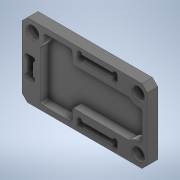
# Autodesk Inventor part: Cockpit_horizontal_frame_06
Saved by Autodesk Inventor 2020 (Build 240168000, 168)
## iProperties
Created: 2021-08-14
Part Number: Cockpit_horizontal_frame_06
Material: アセタール樹脂、黒
Document SubType Name: Modeling
Designer: Masato
Density: 1.425 g/cm^3
Appearance: 滑らか - 黒
Mass: 7.86831 g
Surface Area: 61.8804 cm^2
Volume: 5.52162 cm^3
d0: 59.500 mm
d1: 35.000 mm
d4: 18.833 mm
d6: 18.833 mm
d7: 0.050 mm
d8: 0.050 mm
d9: 1.050 mm
d15: 5.000 mm
d16: 0.00 deg
d17: 2.000 mm
d18: 0.00 deg
d23: 2.500 mm
d26: 35.750 mm
d27: 5.000 mm
d31: 3.200 mm
d32: 6.000 mm
d33: 5.000 mm
d34: 10.000 mm
Author: Masato
Autodesk Inventor part; units mm, degrees
ref_plane "YZ Plane" through (0, 0, 0) normal (1, 0, 0) x (0, 1, 0)
ref_plane "XZ Plane" through (0, 0, 0) normal (0, 1, 0) x (-1, 0, 0)
ref_plane "XY Plane" through (0, 0, 0) normal (0, 0, 1) x (1, 0, 0)
sketch "スケッチ1" plane through (0, 0, 0) normal (0, 0, 1) x (1, 0, 0)
  line L0 (29.75, 17.5) -> (29.75, -17.5)
  line L1 (29.75, -17.5) -> (-29.75, -17.5)
  line L2 (-29.75, -17.5) -> (-29.75, 17.5)
  line L3 (-29.75, 17.5) -> (29.75, -17.5) construction
  line L4 (29.75, 17.5) -> (-29.75, -17.5) construction
  line L5 (-3.4667, -15.05) -> (-1.3667, -15.05) construction
  line L6 (15.4667, -15.05) -> (15.4667, -12.45)
  line L7 (15.4667, -12.45) -> (13.3667, -12.45) construction
  line L8 (-3.4667, -12.45) -> (-3.4667, -15.05)
  line L9 (-3.4667, -15.05) -> (15.4667, -12.45) construction
  line L10 (15.4667, -15.05) -> (-3.4667, -12.45) construction
  line L11 (-3.4167, -12.5) -> (15.4167, -12.5) construction
  line L12 (15.4167, -12.5) -> (15.4167, -15) construction
  line L13 (15.4167, -15) -> (-3.4167, -15) construction
  line L14 (-3.4167, -15) -> (-3.4167, -12.5) construction
  line L15 (-3.4167, -12.5) -> (15.4167, -15) construction
  line L16 (15.4167, -12.5) -> (-3.4167, -15) construction
  arc A0 (-1.3667, -12.45) -> (-3.4667, -12.45) centre (-2.4167, -12.45) ccw
  line L17 (-3.4667, -13.75) -> (15.4667, -13.75) construction
  arc A1 (-3.4667, -15.05) -> (-1.3667, -15.05) centre (-2.4167, -15.05) ccw
  line L18 (-1.3667, -12.45) -> (-3.4667, -12.45) construction
  line L19 (-1.3667, -15.05) -> (13.3667, -15.05)
  line L20 (13.3667, -12.45) -> (-1.3667, -12.45)
  line L21 (13.3667, -15.05) -> (15.4667, -15.05) construction
  line L22 (-29.75, 17.5) -> (29.75, 17.5)
  line L23 (6, 17.5) -> (6, -17.5) construction
  line L24 (-29.75, 0) -> (29.75, 0) construction
  arc A2 (15.4667, -12.45) -> (13.3667, -12.45) centre (14.4167, -12.45) ccw
  arc A3 (13.3667, -15.05) -> (15.4667, -15.05) centre (14.4167, -15.05) ccw
  line L25 (-3.4667, 15.05) -> (-1.3667, 15.05) construction
  line L26 (15.4667, 15.05) -> (15.4667, 12.45)
  line L27 (15.4667, 12.45) -> (13.3667, 12.45) construction
  line L28 (-3.4667, 12.45) -> (-3.4667, 15.05)
  line L29 (-3.4667, 15.05) -> (15.4667, 12.45) construction
  line L30 (15.4667, 15.05) -> (-3.4667, 12.45) construction
  line L31 (-3.4167, 12.5) -> (15.4167, 12.5) construction
  line L32 (15.4167, 12.5) -> (15.4167, 15) construction
  line L33 (15.4167, 15) -> (-3.4167, 15) construction
  line L34 (-3.4167, 15) -> (-3.4167, 12.5) construction
  line L35 (-3.4167, 12.5) -> (15.4167, 15) construction
  line L36 (15.4167, 12.5) -> (-3.4167, 15) construction
  arc A4 (-3.4667, 12.45) -> (-1.3667, 12.45) centre (-2.4167, 12.45) ccw
  line L37 (-3.4667, 13.75) -> (15.4667, 13.75) construction
  arc A5 (-1.3667, 15.05) -> (-3.4667, 15.05) centre (-2.4167, 15.05) ccw
  line L38 (-1.3667, 12.45) -> (-3.4667, 12.45) construction
  line L39 (-1.3667, 15.05) -> (13.3667, 15.05)
  line L40 (13.3667, 12.45) -> (-1.3667, 12.45)
  line L41 (13.3667, 15.05) -> (15.4667, 15.05) construction
  arc A6 (15.4667, 15.05) -> (13.3667, 15.05) centre (14.4167, 15.05) ccw
  arc A7 (13.3667, 12.45) -> (15.4667, 12.45) centre (14.4167, 12.45) ccw
  circle A8 centre (25.4167, -12.5) radius 1.6
  circle A9 centre (25.4167, -12.5) radius 3
  circle A10 centre (25.4167, 12.5) radius 1.6
  circle A11 centre (25.4167, 12.5) radius 3
  circle A12 centre (-24.75, 12.5) radius 1.6
  circle A13 centre (-24.75, 12.5) radius 3
  line L42 (-5.9667, -15) -> (-5.9667, -8.9)
  line L43 (-5.9667, -8.9) -> (21.2585, -8.9)
  line L44 (27.25, -7.3146) -> (27.25, 7.3146)
  line L45 (-19.851, 15) -> (-5.9167, 15)
  arc A14 (-21.15, 8.3419) -> (-19.851, 15) centre (-24.75, 12.5) ccw
  line L46 (-27.25, 2.5) -> (-24.75, 2.5) construction
  line L47 (-24.75, 2.5) -> (-24.75, -7.5) construction
  line L48 (-24.75, -7.5) -> (-27.25, -7.5) construction
  line L49 (-27.25, -7.5) -> (-27.25, 2.5) construction
  line L50 (-27.25, 2.5) -> (-24.75, -7.5) construction
  line L51 (-24.75, 2.5) -> (-27.25, -7.5) construction
  line L52 (-27.3, 2.55) -> (-24.7, 2.55)
  line L53 (-24.7, 2.55) -> (-24.7, -7.55)
  line L54 (-24.7, -7.55) -> (-27.3, -7.55)
  line L55 (-27.3, -7.55) -> (-27.3, 2.55)
  line L56 (-27.3, 2.55) -> (-24.7, -7.55) construction
  line L57 (-24.7, 2.55) -> (-27.3, -7.55) construction
  arc A15 (-27.3, 2.55) -> (-27.3, 0.45) centre (-27.3, 1.5) ccw
  line L58 (-26, 2.55) -> (-26, -7.55) construction
  line L59 (-27.3, -2.5) -> (-24.7, -2.5) construction
  arc A16 (-24.7, 0.45) -> (-24.7, 2.55) centre (-24.7, 1.5) ccw
  arc A17 (-27.3, -5.45) -> (-27.3, -7.55) centre (-27.3, -6.5) ccw
  arc A18 (-24.7, -7.55) -> (-24.7, -5.45) centre (-24.7, -6.5) ccw
  line L60 (-21.15, 8.3419) -> (-21.15, -15)
  line L61 (-5.9667, 15) -> (-5.9667, 8.9)
  line L62 (-21.15, -15) -> (-5.9667, -15)
  arc A19 (27.25, -7.3146) -> (21.2585, -8.9) centre (25.4167, -12.5) ccw
  line L63 (-5.9667, 8.9) -> (21.2585, 8.9)
  arc A20 (21.2585, 8.9) -> (27.25, 7.3146) centre (25.4167, 12.5) ccw
  point P0 (0, 0)
  point P1 (6, -13.75)
  point P2 (6, -13.75)
  point P3 (6, -13.75)
  point P4 (6, 13.75)
  point P5 (6, 13.75)
  point P6 (6, 13.75)
  point P7 (-26, -2.5)
  point P8 (-27.3, -5.45)
  point P9 (-24.7, 0.45)
  point P10 (-24.7, -5.45)
  point P11 (-5.9667, 15)
  point P12 (27.25, 7.3146)
  dimension "d0" = 59.5
  dimension "d1" = 35
  dimension "d6" = 18.8333
  dimension "d7" = 0.05
  dimension "d8" = 0.05
  dimension "d9" = 1.05
  dimension "d26" = 35.75
  dimension "d27" = 5
  dimension "d31" = 3.2
  dimension "d32" = 6
  dimension "d33" = 5
  dimension "d34" = 10
  dimension "d39" = 5
  dimension "d40" = 5
  dimension "d41" = 3.2
  dimension "d42" = 6
  dimension "d43" = 2.5
  dimension "d50" = 2.5
  dimension "d51" = 2.5
  dimension "d54" = 2.5
  dimension "d56" = 2.5
  dimension "d60" = 1.05
  dimension "d61" = 0.05
  dimension "d62" = 0.05
  dimension "d63" = 2.5
  dimension "d64" = 2.5
  dimension "d65" = 10
  dimension "d68" = 2.5
  dimension "d71" = 2.5
  dimension "d75" = 10
  dimension "d76" = 2.5
  dimension "d77" = 2.5
  constraints: 124 end point, 38 symmetric about line, 30 point on circle, 22 midpoint, 21 centre point, 17 parallel, 12 perpendicular, 7 horizontal, 7 point on line, 5 coincident, 1 vertical, 22 other
  measures "d0" distance of L0.end L1.end
  measures "d1" distance of L1.end L2.end
  measures "d6" distance of L11.start L11.end
  measures "d7" distance between parallel lines of L7 L11
  measures "d8" distance between parallel lines of L8 L14
  measures "d9" radius of A0
  measures "d26" distance between parallel lines of L2 L23
  measures "d27" distance between parallel lines of L1 L11
  measures "d31" diameter of A8
  measures "d32" diameter of A9
  measures "d33" vertical distance of L0.end A8.centre
  measures "d34" distance from line of L12 A8.centre
  measures "d39" horizontal distance of L2.end A12.centre
  measures "d40" horizontal distance of L2.end A12.centre
  measures "d41" diameter of A12
  measures "d42" diameter of A13
  measures "d43" distance of L13.end L11.start
  measures "d50" radial gap between concentric circles of A14 A13
  measures "d51" distance between parallel lines of L45 L22
  measures "d54" distance between parallel lines of L0 L44
  measures "d56" distance edge to line of A0 L43
  measures "d60" radius of A15
  measures "d61" distance from line of L46 L58.start
  measures "d62" distance from line of L49 L59.start
  measures "d63" distance between parallel lines of L47 L49
  measures "d64" distance from line of L24.start L49
  measures "d65" distance between parallel lines of L46 L48
  measures "d68" distance edge to line of A18 L60
  measures "d71" distance from line of L17.start L42
  measures "d75" distance from line of L46 A12.centre
  measures "d76" distance between parallel lines of L1 L62
  measures "d77" radial gap between concentric circles of A9 A19
extrude "押し出し1" add sketch "スケッチ1" along normal blind 5 contours L0 L1 L2 L22
extrude "押し出し2" add sketch "スケッチ1" along normal blind 2 contours A9 | A11 | A13
chamfer "面取り1" distance 2.5 angle 45 4 edges at (-29.75, 17.5, 2.5) (-29.75, -17.5, 2.5) (29.75, 17.5, 2.5) (29.75, -17.5, 2.5)
extrude "押し出し3" add sketch "スケッチ1" along normal blind 1 contours L62 L60 A14 L45 L61 L63 A20 L44 A19 L43 L42
fillet "フィレット1" radius 1 11 edges at (-19.851, 15, 3) (-21.15, 8.3419, 3) (-5.9667, -8.9, 3) (-5.9667, 15, 3) (-5.9667, -15, 3) (-21.15, -15, 3) (21.2585, 8.9, 3) (27.25, 7.3146, 3) (27.25, -7.3146, 3) (21.2585, -8.9, 3) (-5.9667, 8.9, 3)
equation "\"d6\" = d4"
equation "\"d8\" = d7"
equation "\"d41\" = d31"
equation "\"d42\" = d32"
equation "\"d50\" = d49"
equation "\"d60\" = d9"
equation "\"d61\" = d7"
equation "\"d62\" = d61"
equation "\"d4\" = 18.833333"
equation "\"d49\" = 2.5"
